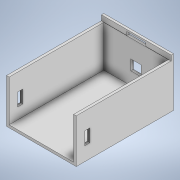
# Autodesk Inventor part: bin v1
Saved by Autodesk Inventor 2022.2 (Build 262287000, 287)
## iProperties
Created: 2022-01-24
Part Number: bin v1
Material: Generic
Document SubType Name: Modeling
Designer: samlo
Density: 1 g/cm^3
Appearance: Default
Author: samlo
Autodesk Inventor part; units mm, degrees
ref_plane "YZ Plane" through (0, 0, 0) normal (1, 0, 0) x (0, 1, 0)
ref_plane "XZ Plane" through (0, 0, 0) normal (0, 1, 0) x (-1, 0, 0)
ref_plane "XY Plane" through (0, 0, 0) normal (0, 0, 1) x (1, 0, 0)
sketch "Sketch1" plane through (0, 0, 0) normal (0, 1, 0) x (-1, 0, 0)
  line L0 (0, 0) -> (81, 0)
  line L1 (81, 0) -> (81, -116)
  line L2 (81, -116) -> (0, -116)
  line L3 (0, -116) -> (0, 0)
  dimension "d0" = 81
  dimension "d1" = 116
  constraints: 8 end point, 2 parallel, 1 horizontal, 1 perpendicular
  measures "d0" distance of L1.end L2.end
  measures "d1" distance of L2.end L0.start
extrude "Extrusion1" add sketch "Sketch1" along normal blind 3
sketch "Sketch2" plane through (0, 3, 0) normal (0, 1, 0) x (1, 0, 0)
  line L0 (0, 116) -> (-81, 116) projected
  line L1 (0, 0) -> (-81, 0)
  line L2 (-81, 0) -> (-81, 116)
  line L3 (-81, 116) -> (0, 116)
  line L4 (0, 116) -> (0, 0)
  line L5 (-3, 3) -> (-78, 3)
  line L6 (-78, 3) -> (-78, 113)
  line L7 (-78, 113) -> (-3, 113)
  line L8 (-3, 113) -> (-3, 3)
  dimension "d4" = 3
  dimension "d5" = 3
  dimension "d6" = 3
  dimension "d7" = 3
  constraints: 16 end point, 4 parallel, 2 horizontal, 2 perpendicular
  measures "d4" distance between parallel lines of L8 L4
  measures "d5" distance between parallel lines of L1 L5
  measures "d6" distance between parallel lines of L7 L0
  measures "d7" distance between parallel lines of L2 L6
extrude "Extrusion2" add sketch "Sketch2" along normal blind 48
sketch "Sketch3" plane through (-81, 0, 0) normal (0, 0, 1) x (1, 0, 0)
  line L0 (0, 51) -> (81, 51) projected
  line L1 (0, 51) -> (81, 51)
  line L2 (81, 51) -> (81, 0)
  line L3 (81, 0) -> (0, 0)
  line L4 (0, 0) -> (0, 51)
  constraints: 8 end point, 2 parallel, 1 horizontal, 1 perpendicular
extrude "Extrusion3" cut sketch "Sketch3" against normal up to surface (3 mm away)
sketch "Sketch4" plane through (0, 51, 0) normal (0, 1, 0) x (1, 0, 0)
  line L0 (-81, 116) -> (-81, 3) projected
  line L1 (0, 3) -> (0, 116) projected
  line L2 (-81, 116) -> (0, 116)
  line L3 (0, 116) -> (0, 113.2852)
  line L4 (0, 113.2852) -> (-81, 113.2852)
  line L5 (-81, 113.2852) -> (-81, 116)
  point P0 (0, 0)
  point P1 (0, 116)
  constraints: 8 end point, 2 parallel, 1 horizontal, 1 perpendicular, 1 point on line
extrude "Extrusion4" add sketch "Sketch4" along normal blind 6
sketch "Sketch5" plane through (0, 0, -116) normal (0, 0, -1) x (-1, 0, 0)
  line L0 (29.5, 55) -> (51.5, 55)
  line L1 (51.5, 55) -> (51.5, 51)
  line L2 (51.5, 51) -> (29.5, 51)
  line L3 (29.5, 51) -> (29.5, 55)
  line L4 (34.5, 30) -> (46.5, 30)
  line L5 (46.5, 30) -> (46.5, 18)
  line L6 (46.5, 18) -> (34.5, 18)
  line L7 (34.5, 18) -> (34.5, 30)
  line L8 (81, 0) -> (81, 57) projected
  line L9 (0, 0) -> (81, 0) projected
  line L10 (0, 57) -> (81, 57) projected
  point P0 (51.5, 53)
  dimension "d14" = 12
  dimension "d15" = 12
  dimension "d16" = 34.5
  dimension "d17" = 18
  dimension "d18" = 22
  dimension "d19" = 4
  dimension "d20" = 6
  dimension "d21" = 29.5
  constraints: 16 end point, 4 parallel, 2 horizontal, 2 perpendicular, 1 midpoint
  measures "d14" distance of L5.end L6.end
  measures "d15" distance of L4.end L5.end
  measures "d16" distance between parallel lines of L8 L5
  measures "d17" distance between parallel lines of L9 L6
  measures "d18" distance of L0.start L0.end
  measures "d19" distance of L0.start L2.end
  measures "d20" distance between parallel lines of L10 L2
  measures "d21" distance from line of L8 point (51.5, 53)
extrude "Extrusion5" cut sketch "Sketch5" against normal up to surface (3 mm away)
sketch "Sketch6" plane through (0, 0, -3) normal (1, 0, 0) x (0, 0, -1)
  line L0 (10, 31) -> (16, 31)
  line L1 (16, 31) -> (16, 16)
  line L2 (16, 16) -> (10, 16)
  line L3 (10, 16) -> (10, 31)
  line L4 (0, 51) -> (0, 0) projected
  line L5 (0, 0) -> (113, 0) projected
  point P0 (-3, 0)
  point P1 (13, 16)
  dimension "d24" = 6
  dimension "d25" = 15
  dimension "d26" = 10
  dimension "d27" = 16
  constraints: 8 end point, 2 parallel, 1 horizontal, 1 midpoint, 1 perpendicular
  measures "d24" distance of L1.end L2.end
  measures "d25" distance of L0.start L2.end
  measures "d26" distance between parallel lines of L3 L4
  measures "d27" distance from line of L5 point (13, 16)
extrude "Extrusion6" cut sketch "Sketch6" against normal up to surface (81 mm away)
body "Solid1"
